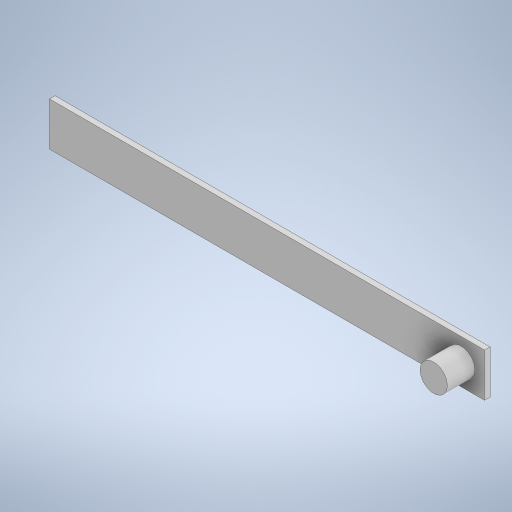
# Autodesk Inventor part: Belt
Saved by Autodesk Inventor 2024 (Build 280153000, 153)
## iProperties
Created: 2024-01-14
Part Number: Belt
Material: Generic
Document SubType Name: Modeling
Designer: Owner
Density: 1 g/cm^3
Appearance: Default
Author: Owner
Autodesk Inventor part; units mm, degrees
ref_plane "YZ Plane" through (0, 0, 0) normal (1, 0, 0) x (0, 1, 0)
ref_plane "XZ Plane" through (0, 0, 0) normal (0, 1, 0) x (-1, 0, 0)
ref_plane "XY Plane" through (0, 0, 0) normal (0, 0, 1) x (1, 0, 0)
sketch "Sketch1" plane through (0, 0, 0) normal (0, 0, 1) x (1, 0, 0)
  line L0 (0, 0) -> (2000, 0)
  line L1 (2000, 0) -> (2000, 200)
  line L2 (2000, 200) -> (0, 200)
  line L3 (0, 200) -> (0, 0)
  dimension "d0" = 2000
  dimension "d1" = 200
  constraints: 8 end point, 2 parallel, 1 horizontal, 1 perpendicular
  measures "d0" distance of L1.end L2.end
  measures "d1" distance of L0.end L1.end
extrude "Extrusion1" add sketch "Sketch1" along normal blind 25.4
sketch "Sketch2" plane through (0, 0, 25.4) normal (0, 0, 1) x (1, 0, 0)
  circle A0 centre (1893.2025, 100) radius 62.8623
  point P0 (0, 0)
  dimension "d4" = 125.7246
  dimension "d5" = 1895.8417
  constraints: 1 centre point
  measures "d4" diameter of A0
  measures "d5" distance of A0.centre point (0, 0)
extrude "Extrusion2" add sketch "Sketch2" along normal blind 127
body "Solid1"
